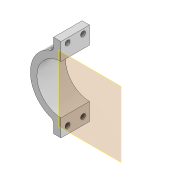
# Autodesk Inventor part: motor mount cap-10
Saved by Autodesk Inventor 2020 (Build 240168000, 168)
## iProperties
Created: 2019-10-28
Part Number: motor mount cap-10
Material: Generic
Document SubType Name: Modeling
Designer: ball
Density: 1 g/cm^3
Appearance: Default
Author: ball
Autodesk Inventor part; units mm, degrees
ref_plane "YZ Plane" through (0, 0, 0) normal (1, 0, 0) x (0, 1, 0)
ref_plane "XZ Plane" through (0, 0, 0) normal (0, 1, 0) x (-1, 0, 0)
ref_plane "XY Plane" through (0, 0, 0) normal (0, 0, 1) x (1, 0, 0)
ref_plane "Work Plane1" through (0, 0, 0) normal (0, 0, 1) x (1, 0, 0)
sketch "Sketch1" plane through (0, 0, 0) normal (0, 0, 1) x (1, 0, 0)
  arc A0 (18.9992, 41.108) -> (0, 60.0877) centre (-0.0008, 41.0877) ccw construction
  arc A1 (0, 22.1284) -> (18.9992, 41.108) centre (-0.0008, 41.1284) ccw construction
  arc A2 (44.3468, 60.0877) -> (25.3476, 41.108) centre (44.3476, 41.0877) ccw construction
  arc A3 (25.3476, 41.108) -> (44.3468, 22.1284) centre (44.3476, 41.1284) ccw construction
  line L0 (10.16, 73.6386) -> (5.7912, 73.6386) construction
  line L1 (0, 77.677) -> (0, 67.7202) construction
  line L2 (5.7912, 73.6386) -> (13.9012, 73.6386) construction
  line L3 (-25.35, 77.677) -> (-25.35, 84.027) projected
  line L4 (-25.35, -6.35) -> (-25.35, 0) projected
  line L5 (-25.35, 77.677) -> (-25.35, 0) construction
  arc A4 (-6.0324, 64.4924) -> (-6.0325, 17.7644) centre (-0.0008, 41.1284) ccw
  arc A5 (-6.0324, 64.4924) -> (-6.0325, 17.7644) centre (-0.0008, 41.1284) ccw
  arc A6 (-0.2548, 60.1259) -> (-0.2548, 22.1309) centre (-0.0008, 41.1284) ccw
  line L6 (-6.0324, 64.4924) -> (-6.0324, 73.6386)
  line L7 (-6.0324, 73.6386) -> (-0.2548, 73.6385)
  line L8 (10.16, 8.5775) -> (5.7912, 8.5775) construction
  line L9 (-6.0325, 8.5775) -> (-0.2548, 8.5775)
  line L10 (-6.0325, 8.5775) -> (-6.0325, 17.7644)
  line L11 (-0.2548, 73.6385) -> (-0.2548, 60.1259)
  line L12 (-0.2548, 8.5775) -> (-0.2548, 22.1309)
  point P0 (0, 0)
  dimension "d12" = 18.9992
  dimension "d13" = 24.13
  dimension "d19" = 6.0317
  dimension "d22" = 6.0317
  dimension "d23" = 0.254
  dimension "d24" = 0.254
  constraints: 16 end point, 7 point on circle, 4 vertical, 3 centre point, 1 coincident, 1 horizontal, 1 point on line
  measures "d12" radius of A6
  measures "d13" radius of A5
  measures "d19" distance from line of L10 A1.centre
  measures "d22" distance from line of L6 A0.centre
  measures "d23" distance from line of L11 A0.centre
  measures "d24" distance from line of L12 A0.centre
ref_plane "Work Plane2" through (0, 17.6708, -22.228) normal (0, 0, -1) x (0, 1, 0)
extrude "Extrusion1" add sketch "Sketch1" against normal up to surface (22.228 mm away)
sketch "Sketch2" plane through (-6.0324, 64.4924, 0) normal (-1, 0.0000012, 0) x (0, 0, 1)
  circle A0 centre (-17.148, 5.715) radius 1.9304
  circle A1 centre (-5.08, 5.715) radius 1.9304
  circle A2 centre (-5.08, -50.0243) radius 1.9304
  circle A3 centre (-17.148, -50.0243) radius 1.9304
  point P0 (0, -64.4924)
  constraints: 4 centre point, 8 other
extrude "Extrusion2" cut sketch "Sketch2" along normal mid plane 25.4
fillet "Fillet1" radius 3.175 1 edges at (-6.0324, 64.4924, -11.114)
fillet "Fillet2" radius 3.175 1 edges at (-6.0325, 17.7644, -11.114)
equation "\"d19\" = d18"
equation "\"d24\" = d23"
equation "\"d18\" = 6.031656"
body "Solid1"
